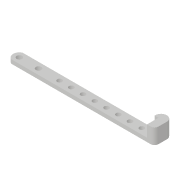
# Autodesk Inventor part: CollectorArmRear
Saved by Autodesk Inventor 2018 (Build 220112000, 112)
## iProperties
Created: 2018-12-27
Part Number: CollectorArmRear
Material: Generic
Document SubType Name: Modeling
Designer: ball
Density: 1 g/cm^3
Appearance: Default
Author: ball
Autodesk Inventor part; units mm, degrees
ref_plane "YZ Plane" through (0, 0, 0) normal (1, 0, 0) x (0, 1, 0)
ref_plane "XZ Plane" through (0, 0, 0) normal (0, 1, 0) x (-1, 0, 0)
ref_plane "XY Plane" through (0, 0, 0) normal (0, 0, 1) x (1, 0, 0)
sketch "Sketch1" plane through (0, 0, 0) normal (0, 1, 0) x (-1, 0, 0)
  line L0 (0, 0) -> (119.38, 0)
  line L1 (119.38, -9.525) -> (9.525, -9.525)
  line L2 (0, -9.525) -> (0, 0)
  arc A0 (0, -9.525) -> (9.525, -9.525) centre (4.7625, -10.16) ccw
  arc A1 (119.38, -9.525) -> (119.38, 0) centre (117.4254, -4.7625) ccw
  circle A2 centre (117.4254, -4.7625) radius 2.2479
  circle A3 centre (101.4234, -4.7625) radius 2.2479
  circle A4 centre (83.872, -4.7625) radius 1.9685
  circle A5 centre (74.093, -4.7625) radius 1.9685
  circle A6 centre (64.314, -4.7625) radius 1.9685
  circle A7 centre (54.535, -4.7625) radius 1.9685
  circle A8 centre (44.756, -4.7625) radius 1.9685
  circle A9 centre (34.977, -4.7625) radius 1.9685
  circle A10 centre (25.198, -4.7625) radius 1.9685
  circle A11 centre (15.419, -4.7625) radius 1.9685
  dimension "d9" = 9.525
  dimension "d10" = 119.38
  dimension "d11" = 4.4958
  dimension "d12" = 4.4958
  dimension "d13" = 16.002
  dimension "d14" = 3.937
  dimension "d15" = 17.5514
  dimension "d18" = 9.779
  constraints: 12 centre point, 6 end point, 4 point on circle, 2 horizontal, 1 coincident, 1 parallel, 14 other
  measures "d9" distance between parallel lines of L0 L1
  measures "d10" distance from line of L2 L0.end
  measures "d11" diameter of A2
  measures "d12" diameter of A3
  measures "d13" distance of A3.centre A1.centre
  measures "d14" diameter of A4
  measures "d15" distance of A4.centre A3.centre
  measures "d18" distance of A4.centre A5.centre
extrude "Extrusion1" add sketch "Sketch1" along normal blind 3.175
sketch "Sketch2" plane through (0, 3.175, 0) normal (0, 1, 0) x (1, 0, 0)
  circle A0 centre (-34.977, 4.7625) radius 1.9685 construction
  arc A1 (0, 9.525) -> (-9.525, 9.525) centre (-4.7625, 10.16) ccw construction
  line L0 (0, 0) -> (-6.35, 0)
  line L1 (-6.35, 0) -> (-6.35, 9.525)
  line L2 (-9.525, 9.525) -> (-6.35, 9.525)
  line L3 (0, 9.525) -> (0, 0)
  line L4 (-119.38, 0) -> (0, 0) projected
  line L5 (0, 0) -> (0, 9.525) projected
  arc A2 (0, 9.525) -> (-9.525, 9.525) centre (-4.7625, 10.16) ccw
  point P0 (-4.7625, 4.7625)
  dimension "d27" = 0
  dimension "d28" = 6.35
  dimension "d32" = 0
  constraints: 8 end point, 2 parallel, 2 point on circle, 1 centre point, 1 coincident, 1 concentric, 1 horizontal, 1 perpendicular
  measures "d27" distance between parallel lines of L5 L3
  measures "d28" distance between parallel lines of L3 L1
  measures "d32" distance between parallel lines of L4 L0
extrude "Extrusion2" add sketch "Sketch2" along normal blind 9.525
fillet "Fillet2" radius 3.175 1 edges at (0, 6.35, 0)
body "Solid1"
